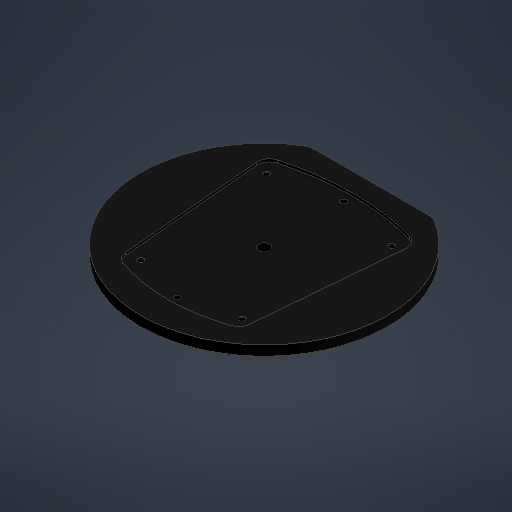
# Autodesk Inventor part: SpiegelabdeckungSSL
Saved by Autodesk Inventor 2025.2 (Build 292293000, 293)
## iProperties
Created: 2025-03-11
Part Number: SpiegelabdeckungSSL
Material: Generisch
Document SubType Name: Modeling
Designer: Faabs
Density: 1 g/cm^3
Appearance: Vorgabe
Author: Faabs
Autodesk Inventor part; units mm, degrees
ref_plane "YZ Plane" through (0, 0, 0) normal (1, 0, 0) x (0, 1, 0)
ref_plane "XZ Plane" through (0, 0, 0) normal (0, 1, 0) x (-1, 0, 0)
ref_plane "XY Plane" through (0, 0, 0) normal (0, 0, 1) x (1, 0, 0)
sketch "Skizze1" plane through (0, 0, 0) normal (0, 0, 1) x (1, 0, 0)
  arc A0 (-47.2504, 56.6131) -> (-53.0963, 48.2064) centre (-45.1265, 48.9002) ccw
  arc A1 (47.2504, 56.6131) -> (-47.2504, 56.6131) centre (0, -114.9743) ccw
  arc A2 (53.0963, 48.2064) -> (47.2504, 56.6131) centre (45.1265, 48.9002) ccw
  line L0 (53.0963, 48.2064) -> (44.103, -55.104)
  arc A3 (38.7321, -61.9763) -> (44.103, -55.104) centre (36.1331, -54.4103) ccw
  arc A4 (-38.7321, -61.9763) -> (38.7321, -61.9763) centre (0, 50.7799) ccw
  arc A5 (-44.103, -55.104) -> (-38.7321, -61.9763) centre (-36.1331, -54.4103) ccw
  line L1 (-44.103, -55.104) -> (-53.0963, 48.2064)
  circle A6 centre (0, -62.4432) radius 1.6
  circle A7 centre (0, 57) radius 1.6
  circle A8 centre (-44.9364, 46.717) radius 2.1
  circle A9 centre (-36.329, -52.1602) radius 2.1
  circle A10 centre (0, 0) radius 2.1
  circle A11 centre (44.9364, 46.717) radius 2.1
  circle A12 centre (36.329, -52.1602) radius 2.1
  circle A13 centre (-44.9364, 46.717) radius 4
  circle A14 centre (44.9364, 46.717) radius 4
  circle A15 centre (36.329, -52.1602) radius 4
  circle A16 centre (-36.329, -52.1602) radius 4
  circle A17 centre (0, -62.4432) radius 3.5
  circle A18 centre (0, 57) radius 3.5
  circle A19 centre (0, 0) radius 20
  arc A20 (-46.1884, 52.7567) -> (-49.1114, 48.5533) centre (-45.1265, 48.9002) ccw
  line L2 (-49.1114, 48.5533) -> (-40.118, -54.7572)
  arc A21 (-40.118, -54.7572) -> (-37.4326, -58.1933) centre (-36.1331, -54.4103) ccw
  arc A22 (-37.4326, -58.1933) -> (37.4326, -58.1933) centre (0, 50.7799) ccw
  arc A23 (37.4326, -58.1933) -> (40.118, -54.7572) centre (36.1331, -54.4103) ccw
  line L3 (40.118, -54.7572) -> (49.1114, 48.5533)
  arc A24 (49.1114, 48.5533) -> (46.1884, 52.7567) centre (45.1265, 48.9002) ccw
  arc A25 (46.1884, 52.7567) -> (-46.1884, 52.7567) centre (0, -114.9743) ccw
  circle A26 centre (0, 0) radius 24
  point P0 (0, 0)
  point P1 (-2.8888, 58.976)
  point P2 (2.8888, 58.976)
  point P3 (2.8973, -64.4067)
  point P4 (-2.8973, -64.4067)
  dimension "d0" = 8
  dimension "d1" = 8
  dimension "d2" = 8
  dimension "d3" = 8
  dimension "d4" = 7
  dimension "d5" = 7
  dimension "d6" = 40
  dimension "d7" = 4
  dimension "d8" = 4
  constraints: 27 centre point, 24 point on circle, 8 coincident, 8 end point, 7 other
  measures "d0" diameter of A13
  measures "d1" diameter of A14
  measures "d2" diameter of A15
  measures "d3" diameter of A16
  measures "d4" diameter of A17
  measures "d5" diameter of A18
  measures "d6" diameter of A19
  measures "d7" radial gap between concentric circles of A1 A25
  measures "d8" radial gap between concentric circles of A19 A26
extrude "Extrusion1" add sketch "Skizze1" against normal blind 5 contours A1 A2 L0 A3 A4 A5 L1 A0 | L2 A20 A25 A18 A24 L3 A23 A22 A17 A21 | A25 A18 | A18 A25 | A22 A17 | A17 A22 | A19 | A26
sketch "Skizze2" plane through (0, 0, -5) normal (0, 0, -1) x (-1, 0, 0)
  circle A0 centre (0, 0) radius 26
  circle A1 centre (54.772, 35) radius 21
  circle A2 centre (54.772, 35) radius 21
  circle A3 centre (-54.772, 35) radius 21
  circle A4 centre (-54.772, 35) radius 21
  circle A5 centre (-35, -54.772) radius 21
  circle A6 centre (-35, -54.772) radius 21
  circle A7 centre (35, -54.772) radius 21
  circle A8 centre (35, -54.772) radius 21
  arc A9 (-44.0306, 77) -> (44.0306, 77) centre (0, 0) ccw
  line L0 (-29, 77) -> (-44.0306, 77)
  line L1 (-44.0306, 77) -> (44.0306, 77)
  circle A10 centre (44.9364, 46.717) radius 4 projected
  circle A11 centre (-44.9364, 46.717) radius 4 projected
  circle A12 centre (-36.329, -52.1602) radius 4 projected
  circle A13 centre (36.329, -52.1602) radius 4 projected
  circle A14 centre (0, -62.4432) radius 1.6 projected
  circle A15 centre (0, 57) radius 1.6 projected
  arc A16 (53.0963, 48.2064) -> (47.2504, 56.6131) centre (45.1265, 48.9002) ccw projected
  line L2 (53.0963, 48.2064) -> (44.103, -55.104) projected
  arc A17 (38.7321, -61.9763) -> (44.103, -55.104) centre (36.1331, -54.4103) ccw projected
  arc A18 (-38.7321, -61.9763) -> (38.7321, -61.9763) centre (0, 50.7799) ccw projected
  arc A19 (-44.103, -55.104) -> (-38.7321, -61.9763) centre (-36.1331, -54.4103) ccw projected
  line L3 (-44.103, -55.104) -> (-53.0963, 48.2064) projected
  arc A20 (-47.2504, 56.6131) -> (-53.0963, 48.2064) centre (-45.1265, 48.9002) ccw projected
  arc A21 (47.2504, 56.6131) -> (-47.2504, 56.6131) centre (0, -114.9743) ccw projected
  circle A22 centre (0, 0) radius 2.1 projected
  constraints: 10 centre point, 6 coincident, 4 end point, 2 point on circle
extrude "Extrusion3" add sketch "Skizze2" against normal blind 5 contours A1 L2 A16 | A7 A18 A17 L2 | A20 L3 A3 | A5 L3 A19 A18 | L0 L1 A9 picked at (55.8063, 25.5813) picked at (36.6001, -67.1417) picked at (-56.1388, 25.6369) picked at (-36.8762, -67.0802)
sketch "Skizze5" plane through (0, 0, 0) normal (0, 0, 1) x (1, 0, 0)
  circle A0 centre (0, 0) radius 20
  circle A1 centre (44.9364, 46.717) radius 4
  circle A2 centre (-44.9364, 46.717) radius 4
  circle A3 centre (-36.329, -52.1602) radius 4
  circle A4 centre (36.329, -52.1602) radius 4
  circle A5 centre (0, -62.4432) radius 1.6
  circle A6 centre (0, 57) radius 1.6
  arc A7 (53.0963, 48.2064) -> (47.2504, 56.6131) centre (45.1265, 48.9002) ccw
  line L0 (53.0963, 48.2064) -> (44.103, -55.104)
  arc A8 (38.7321, -61.9763) -> (44.103, -55.104) centre (36.1331, -54.4103) ccw
  arc A9 (-38.7321, -61.9763) -> (38.7321, -61.9763) centre (0, 50.7799) ccw
  arc A10 (-44.103, -55.104) -> (-38.7321, -61.9763) centre (-36.1331, -54.4103) ccw
  line L1 (-44.103, -55.104) -> (-53.0963, 48.2064)
  arc A11 (-47.2504, 56.6131) -> (-53.0963, 48.2064) centre (-45.1265, 48.9002) ccw
  arc A12 (47.2504, 56.6131) -> (-47.2504, 56.6131) centre (0, -114.9743) ccw
  arc A13 (-47.3832, 57.0952) -> (-53.5945, 48.1631) centre (-45.1265, 48.9002) ccw
  line L2 (-53.5945, 48.1631) -> (-44.6011, -55.1474)
  arc A14 (-44.6011, -55.1474) -> (-38.8945, -62.4492) centre (-36.1331, -54.4103) ccw
  arc A15 (-38.8945, -62.4492) -> (38.8945, -62.4492) centre (0, 50.7799) ccw
  arc A16 (38.8945, -62.4492) -> (44.6011, -55.1474) centre (36.1331, -54.4103) ccw
  line L3 (44.6011, -55.1474) -> (53.5945, 48.1631)
  arc A17 (53.5945, 48.1631) -> (47.3832, 57.0952) centre (45.1265, 48.9002) ccw
  arc A18 (47.3832, 57.0952) -> (-47.3832, 57.0952) centre (0, -114.9743) ccw
  dimension "d19" = 0.5
  constraints: 24 point on circle, 19 centre point, 8 end point, 7 other
  measures "d19" radial gap between concentric circles of A12 A18
extrude "Extrusion5" cut sketch "Skizze5" against normal blind 2 contours A0 | A1 | A2 | A3 | A4 | A5 | A6 | L0 A8 A9 A10 L1 A11 A12 A7 | A18 A17 L3 A16 A15 A14 L2 A13
sketch "Skizze6" plane through (0, 0, -5) normal (0, 0, -1) x (-1, 0, 0)
  arc A0 (-44.0306, 77) -> (44.0306, 77) centre (0, 0) ccw projected
  line L0 (-44.0306, 77) -> (44.0306, 77) projected
  circle A1 centre (44.9364, 46.717) radius 4 projected
  circle A2 centre (-44.9364, 46.717) radius 4 projected
  circle A3 centre (-36.329, -52.1602) radius 4 projected
  circle A4 centre (36.329, -52.1602) radius 4 projected
  circle A5 centre (0, -62.4432) radius 1.6 projected
  circle A6 centre (0, 57) radius 1.6 projected
  circle A7 centre (0, 0) radius 2.1 projected
  circle A8 centre (36.329, -52.1602) radius 7.5
  circle A9 centre (-36.329, -52.1602) radius 7.5
  circle A10 centre (-44.9364, 46.717) radius 7.5
  circle A11 centre (44.9364, 46.717) radius 7.5
  dimension "d37" = 15
  dimension "d38" = 15
  dimension "d39" = 15
  dimension "d40" = 15
  constraints: 4 centre point, 4 coincident
  measures "d37" diameter of A8
  measures "d38" diameter of A9
  measures "d39" diameter of A10
  measures "d40" diameter of A11
extrude "Extrusion6" add sketch "Skizze6" along normal blind 4 contours L0 A0 | A7
sketch "Skizze7" plane through (0, 0, -9) normal (0, 0, -1) x (-1, 0, 0)
  circle A0 centre (0, 0) radius 4
  circle A1 centre (0, 0) radius 20 projected
  circle A2 centre (0, 0) radius 2.1
  dimension "d24" = 8
  dimension "d31" = 4.2
  constraints: 2 centre point, 2 coincident
  measures "d24" diameter of A0
  measures "d31" diameter of A2
sketch "Skizze8" plane through (0, 0, -2) normal (0, 0, 1) x (1, 0, 0)
  circle A0 centre (-44.9364, 46.717) radius 4 projected
  circle A1 centre (-44.9364, 46.717) radius 4
  circle A2 centre (44.9364, 46.717) radius 4 projected
  circle A3 centre (44.9364, 46.717) radius 4
  circle A4 centre (36.329, -52.1602) radius 4 projected
  circle A5 centre (36.329, -52.1602) radius 4
  circle A6 centre (-36.329, -52.1602) radius 4 projected
  circle A7 centre (-36.329, -52.1602) radius 4
  circle A8 centre (-44.9364, 46.717) radius 2.1
  circle A9 centre (44.9364, 46.717) radius 2.1
  circle A10 centre (36.329, -52.1602) radius 2.1
  circle A11 centre (-36.329, -52.1602) radius 2.1
  point P0 (0, 0)
  dimension "d25" = 4.2
  dimension "d26" = 4.2
  dimension "d27" = 4.2
  dimension "d28" = 4.2
  constraints: 8 centre point, 8 coincident
  measures "d25" diameter of A8
  measures "d26" diameter of A9
  measures "d27" diameter of A10
  measures "d28" diameter of A11
extrude "Extrusion7" add sketch "Skizze8" against normal blind 1
extrude "Extrusion8" cut sketch "Skizze7" against normal up to surface (4 mm away) contours A2
sketch "Skizze9" plane through (0, 0, -2) normal (0, 0, 1) x (1, 0, 0)
  circle A0 centre (0, 0) radius 2.1 projected
  circle A1 centre (0, 0) radius 4
  dimension "d34" = 8
  constraints: 1 centre point, 1 coincident
  measures "d34" diameter of A1
extrude "Extrusion9" cut sketch "Skizze9" against normal up to surface (7 mm away) contours A0 | A1
sketch "Skizze10" plane through (-36.329, -52.1602, -5) normal (0, 0, -1) x (-1, 0, 0)
  circle A0 centre (0, 0) radius 2.1 projected
  circle A1 centre (0, 0) radius 4
  circle A2 centre (0, 0) radius 7.5
  circle A3 centre (-72.6579, 0) radius 2.1 projected
  circle A4 centre (-81.2654, 98.8771) radius 2.1 projected
  circle A5 centre (8.6075, 98.8771) radius 2.1 projected
  circle A6 centre (-72.6579, 0) radius 4
  circle A7 centre (-72.6579, 0) radius 7.5
  circle A8 centre (-81.2654, 98.8771) radius 4
  circle A9 centre (-81.2654, 98.8771) radius 7.5
  circle A10 centre (8.6075, 98.8771) radius 4
  circle A11 centre (8.6075, 98.8771) radius 7.5
  point P0 (-36.329, 52.1602)
  constraints: 8 centre point, 8 coincident
extrude "Extrusion10" cut sketch "Skizze10" against normal up to surface (2 mm away) contours A2 | A7 | A9 | A11
fillet "Rundung2" radius 10 2 edges at (44.0306, 77, -4.5) (-44.0306, 77, -4.5)
sketch "Skizze11" plane through (0, 0, -2) normal (0, 0, 1) x (1, 0, 0)
  circle A0 centre (0, 57) radius 1.6 projected
  circle A1 centre (0, 57) radius 2.1
  circle A2 centre (0, -62.4432) radius 1.6 projected
  circle A3 centre (0, -62.4432) radius 2.1
  point P0 (0, 0)
  dimension "d47" = 4.2
  dimension "d48" = 4.2
  constraints: 2 centre point, 2 coincident
  measures "d47" diameter of A1
  measures "d48" diameter of A3
extrude "Extrusion11" cut sketch "Skizze11" against normal blind 6 contours A0 | A1 | A2 | A3
sketch "Skizze12" plane through (0, 0, -9) normal (0, 0, -1) x (-1, 0, 0)
  circle A0 centre (0, -62.4432) radius 1.6 projected
  circle A1 centre (0, -62.4432) radius 1.6
  circle A2 centre (0, 57) radius 1.6 projected
  circle A3 centre (0, 57) radius 1.6
  point P0 (0, 0)
  constraints: 2 centre point, 2 coincident
extrude "Extrusion12" add sketch "Skizze12" against normal up to surface (1 mm away)
chamfer "Fasen2" distance 2 angle 45 1 edges at (0, -88.7, -9)
